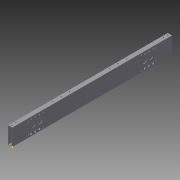
# Autodesk Inventor part: boxbeam 4x1 with sideways holes
Saved by Autodesk Inventor 2015 (Build 190159000, 159)
## iProperties
Created: 2015-01-31
Part Number: boxbeam 4x1 with sideways holes
Material: Generic
Document SubType Name: Modeling
Designer: szymsea16
Density: 1 g/cm^3
Appearance: Default
Author: szymsea16
Autodesk Inventor part; units mm, degrees
ref_plane "YZ Plane" through (0, 0, 0) normal (1, 0, 0) x (0, 1, 0)
ref_plane "XZ Plane" through (0, 0, 0) normal (0, 1, 0) x (-1, 0, 0)
ref_plane "XY Plane" through (0, 0, 0) normal (0, 0, 1) x (1, 0, 0)
sketch "Sketch1" plane through (0, 0, 0) normal (0, 1, 0) x (-1, 0, 0)
  line L0 (0, 0) -> (0, -965.2)
  line L1 (0, -965.2) -> (25.4, -965.2)
  line L2 (0, 0) -> (25.4, 0)
  line L3 (25.4, 0) -> (25.4, -965.2)
  dimension "d0" = 965.2
  dimension "d1" = 25.4
  dimension "d2" = 25.4
  dimension "d3" = 965.2
  constraints: 8 end point, 1 parallel, 1 perpendicular, 1 vertical
  measures "d0" distance of L0.start L0.end
  measures "d1" distance of L0.end L1.end
  measures "d2" distance of L0.start L2.end
  measures "d3" distance of L2.end L1.end
extrude "Extrusion1" add sketch "Sketch1" along normal blind 101.6
sketch "Sketch2" plane through (0, 0, -965.2) normal (0, 0, -1) x (-1, 0, 0)
  line L0 (0, 101.6) -> (25.4, 101.6) projected
  line L1 (22.225, 98.425) -> (3.175, 98.425)
  line L2 (3.175, 98.425) -> (3.175, 3.175)
  line L3 (3.175, 3.175) -> (22.225, 3.175)
  line L4 (22.225, 3.175) -> (22.225, 98.425)
  point P0 (0, 0)
  dimension "d8" = 19.05
  dimension "d9" = 95.25
  dimension "d10" = 19.05
  constraints: 8 end point, 2 perpendicular
  measures "d8" distance of L1.start L1.end
  measures "d9" distance of L1.end L2.end
  measures "d10" distance of L2.end L3.end
extrude "Extrusion2" cut sketch "Sketch2" against normal blind 2540
sketch "Sketch3" plane through (-25.4, 0, -965.2) normal (-1, 0, 0) x (0, 0, 1)
  line L0 (204.7889, -13.1279) -> (93.1507, -4.0762)
  arc A0 (87.3139, 2.253) -> (93.1507, -4.0762) centre (93.6639, 2.253) ccw
  line L1 (87.3139, 2.253) -> (87.3139, 98.4911)
  arc A1 (93.1507, 104.8203) -> (87.3139, 98.4911) centre (93.6639, 98.4911) ccw
  line L2 (93.1507, 104.8203) -> (204.7889, 113.8721)
  line L3 (204.7889, 113.8721) -> (206.4399, 113.8721)
  line L4 (206.4399, -13.1279) -> (206.4399, 113.8721)
  line L5 (206.4399, -13.1279) -> (204.7889, -13.1279)
  circle A2 centre (185.2041, 94.9491) radius 2.0447
  circle A3 centre (96.3041, 12.7801) radius 2.0447
  circle A4 centre (185.2041, 89.1071) radius 2.5527
  circle A5 centre (96.3041, 18.6221) radius 2.5527
  circle A6 centre (113.3221, 89.1071) radius 5.5562
  circle A7 centre (164.1221, 89.1071) radius 5.5562
  circle A8 centre (113.3221, 11.6371) radius 5.5562
  circle A9 centre (126.1759, 50.3721) radius 11.1061
  circle A10 centre (138.7221, 11.6371) radius 5.5562
  circle A11 centre (164.1221, 11.6371) radius 5.5562
  circle A12 centre (138.7221, 89.1071) radius 5.5562
  circle A13 centre (166.8921, 50.3721) radius 14.2811
  circle A14 centre (96.3041, 82.1221) radius 2.5527
  circle A15 centre (185.2041, 11.6371) radius 2.5527
  circle A16 centre (96.3041, 87.9641) radius 2.0447
  circle A17 centre (185.2041, 5.7951) radius 2.0447
  circle A18 centre (96.3041, 87.9641) radius 2.0447
  circle A19 centre (96.3041, 82.1221) radius 2.5527
  circle A20 centre (96.3041, 18.6221) radius 2.5527
  circle A21 centre (96.3041, 12.7801) radius 2.0447
  circle A22 centre (126.1759, 50.3721) radius 11.1061
  circle A23 centre (113.3221, 11.6371) radius 5.5563
  circle A24 centre (138.7221, 11.6371) radius 5.5562
  circle A25 centre (164.1221, 11.6371) radius 5.5562
  circle A26 centre (166.8921, 50.3721) radius 14.2811
  circle A27 centre (164.1221, 89.1071) radius 5.5562
  circle A28 centre (138.7221, 89.1071) radius 5.5562
  circle A29 centre (113.3221, 89.1071) radius 5.5562
  circle A30 centre (185.2041, 11.6371) radius 2.5527
  circle A31 centre (185.2041, 5.7951) radius 2.0447
  circle A32 centre (185.2041, 89.1071) radius 2.5527
  circle A33 centre (185.2041, 94.9491) radius 2.0447
  line L6 (759.6672, 114.2512) -> (871.3054, 105.1995)
  arc A34 (877.1422, 98.8702) -> (871.3054, 105.1995) centre (870.7922, 98.8702) ccw
  line L7 (877.1422, 98.8702) -> (877.1422, 2.6322)
  arc A35 (871.3054, -3.697) -> (877.1422, 2.6322) centre (870.7922, 2.6322) ccw
  line L8 (871.3054, -3.697) -> (759.6672, -12.7488)
  line L9 (759.6672, -12.7488) -> (758.0162, -12.7488)
  line L10 (758.0162, 114.2512) -> (758.0162, -12.7488)
  line L11 (758.0162, 114.2512) -> (759.6672, 114.2512)
  circle A36 centre (779.2519, 6.1742) radius 2.0447
  circle A37 centre (868.1519, 88.3432) radius 2.0447
  circle A38 centre (779.2519, 12.0162) radius 2.5527
  circle A39 centre (868.1519, 82.5012) radius 2.5527
  circle A40 centre (851.1339, 12.0162) radius 5.5562
  circle A41 centre (800.3339, 12.0162) radius 5.5562
  circle A42 centre (851.1339, 89.4862) radius 5.5562
  circle A43 centre (838.2802, 50.7512) radius 11.1061
  circle A44 centre (825.7339, 89.4862) radius 5.5562
  circle A45 centre (800.3339, 89.4862) radius 5.5562
  circle A46 centre (825.7339, 12.0162) radius 5.5562
  circle A47 centre (797.564, 50.7512) radius 14.2811
  circle A48 centre (868.1519, 19.0012) radius 2.5527
  circle A49 centre (779.2519, 89.4862) radius 2.5527
  circle A50 centre (868.1519, 13.1592) radius 2.0447
  circle A51 centre (779.2519, 95.3282) radius 2.0447
  circle A52 centre (868.1519, 13.1592) radius 2.0447
  circle A53 centre (868.1519, 19.0012) radius 2.5527
  circle A54 centre (868.1519, 82.5012) radius 2.5527
  circle A55 centre (868.1519, 88.3432) radius 2.0447
  circle A56 centre (838.2802, 50.7512) radius 11.1061
  circle A57 centre (851.1339, 89.4862) radius 5.5563
  circle A58 centre (825.7339, 89.4862) radius 5.5562
  circle A59 centre (800.3339, 89.4862) radius 5.5562
  circle A60 centre (797.564, 50.7512) radius 14.2811
  circle A61 centre (800.3339, 12.0162) radius 5.5562
  circle A62 centre (825.7339, 12.0162) radius 5.5562
  circle A63 centre (851.1339, 12.0162) radius 5.5562
  circle A64 centre (779.2519, 89.4862) radius 2.5527
  circle A65 centre (779.2519, 95.3282) radius 2.0447
  circle A66 centre (779.2519, 12.0162) radius 2.5527
  circle A67 centre (779.2519, 6.1742) radius 2.0447
  line L12 (0, 101.6) -> (0, 50.8)
  line L13 (0, 50.8) -> (127, 50.8)
  line L14 (965.2, 101.6) -> (965.2, 50.8)
  line L15 (965.2, 3.175) -> (965.2, 98.425) projected
  line L16 (965.2, 50.8) -> (838.2, 50.8)
  point P0 (965.2, 0)
  point P1 (106.8311, 102.2108)
  dimension "d13" = 50.8
  dimension "d14" = 127
  dimension "d15" = 50.8
  dimension "d16" = 127
  constraints: 68 centre point, 32 end point, 8 point on circle, 1 horizontal, 1 midpoint, 1 perpendicular
  measures "d13" distance of L12.start L12.end
  measures "d14" distance of L12.end L13.end
  measures "d15" distance of L14.start L14.end
  measures "d16" distance of L14.end L16.end
extrude "Extrusion3" cut sketch "Sketch3" against normal blind 2540 contours A6
extrude "Extrusion4" cut sketch "Sketch3" against normal blind 2540 contours A13
extrude "Extrusion5" cut sketch "Sketch3" against normal blind 2540 contours A7
extrude "Extrusion6" cut sketch "Sketch3" against normal blind 2540 contours A2 | A3 | A4 | A5 | A8 | A9 | A10 | A11 | A12 | A14 | A15 | A16 | A17
extrude "Extrusion7" cut sketch "Sketch3" against normal blind 2540 contours A47
extrude "Extrusion8" cut sketch "Sketch3" against normal blind 2540 contours A36 | A37 | A38 | A39 | A40 | A41 | A42 | A43 | A44 | A45 | A46 | A48 | A49 | A50 | A51
sketch "Sketch5" plane through (0, 0, 0) normal (0, -1, 0) x (1, 0, 0)
  point P0 (0, 0)
body "Solid1"
